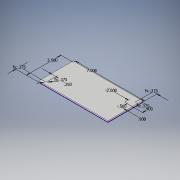
# Autodesk Inventor part: BackCover
Saved by Autodesk Inventor 2018 (Build 220112000, 112)
## iProperties
Created: 2020-03-31
Part Number: BackCover
Material: Generic
Document SubType Name: Modeling
Designer: emile
Density: 1 g/cm^3
Appearance: Default
Author: emile
Autodesk Inventor part; units mm, degrees
ref_plane "YZ Plane" through (0, 0, 0) normal (1, 0, 0) x (0, 1, 0)
ref_plane "XZ Plane" through (0, 0, 0) normal (0, 1, 0) x (-1, 0, 0)
ref_plane "XY Plane" through (0, 0, 0) normal (0, 0, 1) x (1, 0, 0)
sketch "Sketch1" plane through (0, 0, 0) normal (0, 1, 0) x (-1, 0, 0)
  line L0 (-88.9, 44.45) -> (88.9, 44.45)
  line L1 (88.9, 44.45) -> (88.9, -44.45)
  line L2 (88.9, -44.45) -> (-88.9, -44.45)
  line L3 (-88.9, -44.45) -> (-88.9, 44.45)
  line L4 (-88.9, 44.45) -> (88.9, -44.45) construction
  line L5 (88.9, 44.45) -> (-88.9, -44.45) construction
  line L6 (-66.04, -8.89) -> (-15.24, -8.89)
  line L7 (-15.24, -8.89) -> (-15.24, -21.59)
  line L8 (-15.24, -21.59) -> (-66.04, -21.59)
  line L9 (-66.04, -21.59) -> (-66.04, -8.89)
  line L10 (-66.04, -8.89) -> (-15.24, -21.59) construction
  line L11 (-15.24, -8.89) -> (-66.04, -21.59) construction
  point P0 (0, 0)
  point P1 (-40.64, -15.24)
  dimension "d0" = 177.8
  dimension "d1" = 88.9
  dimension "d2" = 22.86
  dimension "d3" = 22.86
  dimension "d4" = 12.7
  dimension "d5" = 50.8
  constraints: 24 end point, 4 midpoint, 4 parallel, 2 horizontal, 2 perpendicular
  measures "d0" distance of L1.end L2.end
  measures "d1" distance of L0.end L1.end
  measures "d2" distance between parallel lines of L2 L8
  measures "d3" distance between parallel lines of L3 L9
  measures "d4" distance of L8.end L6.start
  measures "d5" distance of L7.end L8.end
extrude "Extrusion1" add sketch "Sketch1" along normal blind 3.175 contours L0 L1 L2 L3 | L6 L7 L8 L9
extrude "Extrusion2" add sketch "Sketch1" against normal blind 15.24 contours L6 L7 L8 L9
sketch "Sketch2" plane through (0, 0, 0) normal (0, -1, 0) x (1, 0, 0)
  circle A0 centre (-79.375, 34.925) radius 3.175
  circle A1 centre (-79.375, -34.925) radius 3.175
  circle A2 centre (79.375, 34.925) radius 3.175
  circle A3 centre (79.375, -34.925) radius 3.175
  line L0 (88.9, 44.45) -> (-88.9, 44.45) projected
  line L1 (-88.9, 44.45) -> (-88.9, -44.45) projected
  line L2 (-88.9, -44.45) -> (88.9, -44.45) projected
  line L3 (88.9, -44.45) -> (88.9, 44.45) projected
  point P0 (0, 0)
  dimension "d11" = 9.525
  dimension "d13" = 9.525
  dimension "d14" = 6.35
  dimension "d15" = 9.525
  dimension "d16" = 9.525
  constraints: 4 centre point, 3 equal radius, 2 horizontal alignment, 2 vertical alignment
  measures "d11" distance from line of L1 A0.centre
  measures "d13" distance from line of L3 A3.centre
  measures "d14" diameter of A0
  measures "d15" distance from line of L0 A0.centre
  measures "d16" distance from line of L2 A3.centre
equation "\"d11\" = d10"
equation "\"d13\" = d12"
equation "\"d15\" = d11"
equation "\"d16\" = d13"
equation "\"d12\" = d11"
equation "\"d10\" = 9.525"
body "Solid1"
